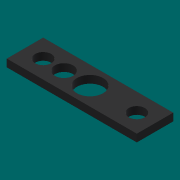
# Autodesk Inventor part: lightGasket
Saved by Autodesk Inventor 2016 (Build 200138000, 138)
## iProperties
Created: 2016-02-15
Part Number: lightGasket
Material: Rubber
Document SubType Name: Modeling
Designer: sawai
Density: 0.93 g/cm^3
Appearance: Rubber - Black
Author: sawai
Autodesk Inventor part; units mm, degrees
ref_plane "YZ Plane" through (0, 0, 0) normal (1, 0, 0) x (0, 1, 0)
ref_plane "XZ Plane" through (0, 0, 0) normal (0, 1, 0) x (-1, 0, 0)
ref_plane "XY Plane" through (0, 0, 0) normal (0, 0, 1) x (1, 0, 0)
sketch "Sketch1" plane through (0, 0, 0) normal (0, 0, 1) x (1, 0, 0)
  line L0 (0, 0) -> (-25, 0)
  line L1 (-25, 0) -> (-25, -7)
  line L2 (-25, -7) -> (0, -7)
  line L3 (0, -7) -> (0, 0)
  circle A0 centre (-21.5, -3.5) radius 1.55
  circle A1 centre (-3.5, -3.5) radius 1.55
  circle A2 centre (-12.5, -3.5) radius 2.525
  circle A3 centre (-17.5, -3.5) radius 1.75
  constraints: 8 end point, 4 centre point
extrude "Extrusion1" add sketch "Sketch1" along normal blind 1.45
body "Solid1"
